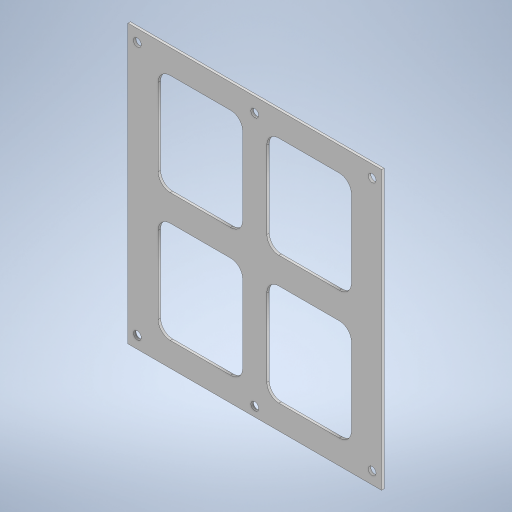
# Autodesk Inventor part: PCB_board_box_top
Saved by Autodesk Inventor 2023 (Build 270158000, 158)
## iProperties
Created: 2023-05-25
Part Number: PCB_board_box_top
Material: 一般
Document SubType Name: Sheet Metal
Designer: 310611102
Density: 1 g/cm^3
Sheet Metal Rule: Default_mm
Appearance: 預設
Author: 310611102
Autodesk Inventor part; units mm, degrees
ref_plane "YZ Plane" through (0, 0, 0) normal (1, 0, 0) x (0, 1, 0)
ref_plane "XZ Plane" through (0, 0, 0) normal (0, 1, 0) x (-1, 0, 0)
ref_plane "XY Plane" through (0, 0, 0) normal (0, 0, 1) x (1, 0, 0)
sketch "Sketch1" plane through (0, 0, 0) normal (0, 0, 1) x (1, 0, 0)
  line L0 (-52.5, 57.5) -> (52.5, 57.5)
  line L1 (52.5, 57.5) -> (52.5, -57.5)
  line L2 (52.5, -57.5) -> (-52.5, -57.5)
  line L3 (-52.5, -57.5) -> (-52.5, 57.5)
  line L4 (-52.5, 57.5) -> (52.5, -57.5) construction
  line L5 (52.5, 57.5) -> (-52.5, -57.5) construction
  line L6 (-35, 47.5) -> (-10, 47.5)
  line L7 (-5, 42.5) -> (-5, 10.5)
  line L8 (-10, 5.5) -> (-35, 5.5)
  line L9 (-40, 10.5) -> (-40, 42.5)
  line L10 (-40, 47.5) -> (-5, 5.5) construction
  line L11 (-5, 47.5) -> (-40, 5.5) construction
  arc A0 (-35, 47.5) -> (-40, 42.5) centre (-35, 42.5) ccw
  arc A1 (-5, 42.5) -> (-10, 47.5) centre (-10, 42.5) ccw
  arc A2 (-10, 5.5) -> (-5, 10.5) centre (-10, 10.5) ccw
  arc A3 (-40, 10.5) -> (-35, 5.5) centre (-35, 10.5) ccw
  line L12 (40, 42.5) -> (40, 10.5)
  line L13 (5, 10.5) -> (5, 42.5)
  arc A4 (40, 42.5) -> (35, 47.5) centre (35, 42.5) ccw
  line L14 (10, 47.5) -> (35, 47.5)
  arc A5 (10, 47.5) -> (5, 42.5) centre (10, 42.5) ccw
  arc A6 (35, 5.5) -> (40, 10.5) centre (35, 10.5) ccw
  line L15 (35, 5.5) -> (10, 5.5)
  arc A7 (5, 10.5) -> (10, 5.5) centre (10, 10.5) ccw
  line L16 (-5, -10.5) -> (-5, -42.5)
  line L17 (-40, -42.5) -> (-40, -10.5)
  arc A8 (-5, -10.5) -> (-10, -5.5) centre (-10, -10.5) ccw
  line L18 (-35, -5.5) -> (-10, -5.5)
  arc A9 (-35, -5.5) -> (-40, -10.5) centre (-35, -10.5) ccw
  arc A10 (-10, -47.5) -> (-5, -42.5) centre (-10, -42.5) ccw
  line L19 (-10, -47.5) -> (-35, -47.5)
  arc A11 (-40, -42.5) -> (-35, -47.5) centre (-35, -42.5) ccw
  line L20 (40, -10.5) -> (40, -42.5)
  line L21 (5, -42.5) -> (5, -10.5)
  arc A12 (40, -10.5) -> (35, -5.5) centre (35, -10.5) ccw
  line L22 (10, -5.5) -> (35, -5.5)
  arc A13 (10, -5.5) -> (5, -10.5) centre (10, -10.5) ccw
  arc A14 (35, -47.5) -> (40, -42.5) centre (35, -42.5) ccw
  line L23 (35, -47.5) -> (10, -47.5)
  arc A15 (5, -42.5) -> (10, -47.5) centre (10, -42.5) ccw
  line L24 (0, 0) -> (0, 8.2827)
  circle A16 centre (-48.6, 52.5) radius 1.6
  line L25 (0, 0) -> (-5.1125, 0)
  circle A17 centre (48.6, 52.5) radius 1.6
  circle A18 centre (-48.6, -52.5) radius 1.6
  circle A19 centre (48.6, -52.5) radius 1.6
  circle A20 centre (0, 51.5) radius 1.6
  circle A21 centre (0, -53.6) radius 1.6
  point P0 (-22.5, 26.5)
  point P1 (22.5, 26.5)
  point P2 (40, 47.5)
  point P3 (40, 5.5)
  point P4 (5, 47.5)
  point P5 (5, 5.5)
  point P6 (-22.5, -26.5)
  point P7 (-5, -5.5)
  point P8 (-5, -47.5)
  point P9 (-40, -5.5)
  point P10 (-40, -47.5)
  point P11 (22.5, -26.5)
  point P12 (40, -5.5)
  point P13 (40, -47.5)
  point P14 (5, -5.5)
  point P15 (5, -47.5)
  point P16 (0, 57.5)
  dimension "d0" = 115
  dimension "d1" = 105
  dimension "d2" = 10
  dimension "d3" = 12.5
  dimension "d4" = 35
  dimension "d5" = 42
  dimension "d6" = 5
  dimension "d9" = 45
  dimension "d12" = 53
  dimension "d18" = 3.2
  dimension "d19" = 5
  dimension "d20" = 3.9
  dimension "d35" = 3.2
  dimension "d37" = 6
  dimension "d39" = 10
  dimension "d40" = 12.5
  dimension "d41" = 11
  dimension "d42" = 10
  dimension "d43" = 3.2
  dimension "d44" = 3.9
  measures "d0" distance of L0.end L1.end
  measures "d1" distance of L0.start L0.end
  measures "d2" distance between parallel lines of L0 L6
  measures "d3" distance between parallel lines of L3 L9
  measures "d4" distance of L10.start L11.start
  measures "d5" distance of L11.start L10.end
  measures "d6" radius of A0
  measures "d9" distance of point (-22.5, 26.5) point (22.5, 26.5)
  measures "d12" distance of point (-22.5, 26.5) point (-22.5, -26.5)
  measures "d18" diameter of A16
  measures "d19" distance from line of L0 A16.centre
  measures "d20" distance from line of L3 A16.centre
  measures "d35" diameter of A20
  measures "d37" distance of point (0, 57.5) A20.centre
  measures "d39" distance between parallel lines of L13 L7
  measures "d40" distance between parallel lines of L1 L12
  measures "d41" distance between parallel lines of L18 L8
  measures "d42" distance between parallel lines of L2 L19
  measures "d43" diameter of A21
  measures "d44" distance from line of L2 A21.centre
sketch "Sketch2" plane through (0, 0, 1) normal (0, 0, 1) x (1, 0, 0)
  arc A0 (27.5, -40) -> (32.5, -35) centre (27.5, -35) ccw
  line L0 (27.5, -40) -> (12.5, -40)
  arc A1 (7.5, -35) -> (12.5, -40) centre (12.5, -35) ccw
  line L1 (7.5, -35) -> (7.5, -10)
  arc A2 (12.5, -5) -> (7.5, -10) centre (12.5, -10) ccw
  line L2 (12.5, -5) -> (27.5, -5)
  arc A3 (32.5, -10) -> (27.5, -5) centre (27.5, -10) ccw
  line L3 (32.5, -10) -> (32.5, -35)
  arc A4 (-7.5, -40) -> (-2.5, -35) centre (-7.5, -35) ccw
  line L4 (-7.5, -40) -> (-22.5, -40)
  arc A5 (-27.5, -35) -> (-22.5, -40) centre (-22.5, -35) ccw
  line L5 (-27.5, -35) -> (-27.5, -10)
  arc A6 (-22.5, -5) -> (-27.5, -10) centre (-22.5, -10) ccw
  line L6 (-22.5, -5) -> (-7.5, -5)
  arc A7 (-2.5, -10) -> (-7.5, -5) centre (-7.5, -10) ccw
  line L7 (-2.5, -10) -> (-2.5, -35)
  arc A8 (27.5, 5) -> (32.5, 10) centre (27.5, 10) ccw
  line L8 (27.5, 5) -> (12.5, 5)
  arc A9 (7.5, 10) -> (12.5, 5) centre (12.5, 10) ccw
  line L9 (7.5, 10) -> (7.5, 35)
  arc A10 (12.5, 40) -> (7.5, 35) centre (12.5, 35) ccw
  line L10 (12.5, 40) -> (27.5, 40)
  arc A11 (32.5, 35) -> (27.5, 40) centre (27.5, 35) ccw
  line L11 (32.5, 35) -> (32.5, 10)
  arc A12 (-22.5, 40) -> (-27.5, 35) centre (-22.5, 35) ccw
  line L12 (-22.5, 40) -> (-7.5, 40)
  arc A13 (-2.5, 35) -> (-7.5, 40) centre (-7.5, 35) ccw
  line L13 (-2.5, 35) -> (-2.5, 10)
  arc A14 (-7.5, 5) -> (-2.5, 10) centre (-7.5, 10) ccw
  line L14 (-7.5, 5) -> (-22.5, 5)
  arc A15 (-27.5, 10) -> (-22.5, 5) centre (-22.5, 10) ccw
  line L15 (-27.5, 10) -> (-27.5, 35)
  circle A16 centre (32.5, -44) radius 1.6
  circle A17 centre (-32.5, -44) radius 1.6
  circle A18 centre (32.5, 44) radius 1.6
  circle A19 centre (-32.5, 44) radius 1.6
  line L16 (37.5, 50) -> (37.5, -50)
  line L17 (-37.5, 50) -> (37.5, 50)
  line L18 (-37.5, -50) -> (-37.5, 50)
  line L19 (37.5, -50) -> (-37.5, -50)
  line L20 (47.5, 60) -> (47.5, -60)
  line L21 (47.5, -60) -> (-47.5, -60)
  line L22 (-47.5, -60) -> (-47.5, 60)
  line L23 (-47.5, 60) -> (47.5, 60)
  circle A20 centre (0, 54) radius 1.6
  circle A21 centre (-41.5, 0) radius 1.6
  line L24 (0, 0) -> (0, 6.9645)
  line L25 (0, 0) -> (5.3167, 0)
  circle A22 centre (0, -54) radius 1.6
  circle A23 centre (41.5, 0) radius 1.6
  dimension "d21" = 10
  dimension "d22" = 3.2
  dimension "d23" = 6
  dimension "d26" = 3.2
  dimension "d29" = 6
  measures "d21" distance between parallel lines of L17 L23
  measures "d22" diameter of A20
  measures "d23" distance from line of L23 A20.centre
  measures "d26" diameter of A21
  measures "d29" distance from line of L22 A21.centre
extrude "Plate1" add sketch "Sketch1" along normal blind 1
equation "\"d15\" = 厚度"
equation "\"折彎半徑\" = 厚度"
equation "\"折彎離隙寬度\" = 厚度"
equation "\"折彎離隙深度\" = 0.5 * 厚度"
equation "\"轉角離隙大小\" = 4 * 厚度"
equation "\"最小剩餘\" = 2 * 厚度"
equation "\"轉移半徑\" = 折彎半徑"
equation "\"Jacobi半徑大小\" = 折彎半徑"
equation "\"間隙大小\" = 厚度"
equation "\"厚度\" = 1"
body "Solid1"
